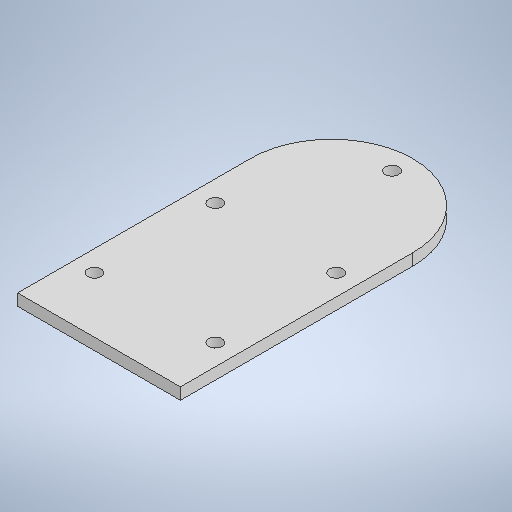
# Autodesk Inventor part: SCARA arm - lid
Saved by Autodesk Inventor 2025.2 (Build 292293000, 293)
## iProperties
Created: 2025-01-29
Part Number: SCARA arm - lid
Material: Generic
Document SubType Name: Modeling
Designer: caomi
Density: 1 g/cm^3
Appearance: Default
Author: caomi
Autodesk Inventor part; units mm, degrees
ref_plane "YZ Plane" through (0, 0, 0) normal (1, 0, 0) x (0, 1, 0)
ref_plane "XZ Plane" through (0, 0, 0) normal (0, 1, 0) x (-1, 0, 0)
ref_plane "XY Plane" through (0, 0, 0) normal (0, 0, 1) x (1, 0, 0)
sketch "Sketch1" plane through (0, 0, 0) normal (0, 1, 0) x (-1, 0, 0)
  line L0 (0, 0) -> (70, 0)
  line L1 (70, 0) -> (70, -100)
  line L2 (70, -100) -> (0, -100)
  line L3 (0, -100) -> (0, 0)
  circle A0 centre (35, -100) radius 35
  point P0 (0, -100)
  dimension "d0" = 70
  dimension "d1" = 100
  constraints: 8 end point, 2 parallel, 1 horizontal, 1 midpoint, 1 perpendicular, 3 other
  measures "d0" distance of L0.start L0.end
  measures "d1" distance of L2.end L0.start
extrude "Extrusion1" add sketch "Sketch1" along normal blind 5
sketch "Sketch2" plane through (0, 5, 0) normal (0, 1, 0) x (1, 0, 0)
  line L0 (-35, -3.9778) -> (-35, 85.9943) construction
  line L1 (-50.1615, 50) -> (-5.6646, 50) construction
  line L2 (-70, 100) -> (-70, 0) projected
  line L3 (-70, 0) -> (0, 0) projected
  arc A0 (0, 100) -> (-70, 100) centre (-35, 100) ccw projected
  point P0 (-61, 24)
  point P1 (-61, 76)
  point P2 (-9, 24)
  point P3 (-9, 76)
  point P4 (-70, 50)
  point P5 (-35, 0)
  point P6 (-35, 126)
  point P7 (-35, 135)
  dimension "d4" = 9
  dimension "d5" = 24
  dimension "d6" = 9
  constraints: 4 end point, 3 point on line, 3 symmetric about line, 2 midpoint, 1 horizontal, 1 point on circle, 1 vertical
  measures "d4" distance from line of L2 point (-61, 24)
  measures "d5" distance from line of L3 point (-61, 24)
  measures "d6" distance of point (-35, 135) point (-35, 126)
hole "Hole1" at (-61, 5, -24) at (-61, 5, -76) at (-9, 5, -24) at (-9, 5, -76) at (-35, 5, -126) direction (0, -1, 0) diameter 4.3 end through all counterbore diameter 5.8 counterbore depth 4
body "Solid1"
